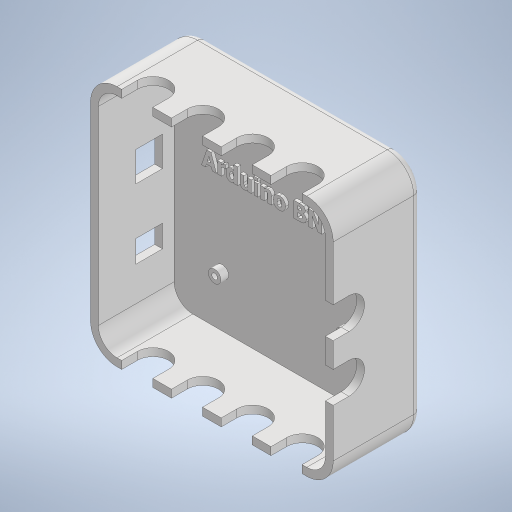
# Autodesk Inventor part: arduino_bnc_case_bottom
Saved by Autodesk Inventor 2024 (Build 280153000, 153)
## iProperties
Created: 2023-07-25
Part Number: arduino_bnc_case_bottom
Material: Generic
Document SubType Name: Modeling
Designer: maimon
Density: 1 g/cm^3
Appearance: Default
Author: maimon
Autodesk Inventor part; units mm, degrees
ref_plane "YZ Plane" through (0, 0, 0) normal (1, 0, 0) x (0, 1, 0)
ref_plane "XZ Plane" through (0, 0, 0) normal (0, 1, 0) x (-1, 0, 0)
ref_plane "XY Plane" through (0, 0, 0) normal (0, 0, 1) x (1, 0, 0)
sketch "Sketch1" plane through (0, 0, 0) normal (0, 0, 1) x (1, 0, 0)
  line L0 (-38.735, -46.355) -> (38.735, -46.355)
  line L1 (46.355, -38.735) -> (46.355, 38.735)
  line L2 (38.735, 46.355) -> (-38.735, 46.355)
  line L3 (-46.355, 38.735) -> (-46.355, -38.735)
  line L4 (-46.355, -46.355) -> (46.355, 46.355) construction
  line L5 (46.355, -46.355) -> (-46.355, 46.355) construction
  arc A0 (-38.735, 46.355) -> (-46.355, 38.735) centre (-38.735, 38.735) ccw
  arc A1 (-46.355, -38.735) -> (-38.735, -46.355) centre (-38.735, -38.735) ccw
  arc A2 (38.735, -46.355) -> (46.355, -38.735) centre (38.735, -38.735) ccw
  arc A3 (46.355, 38.735) -> (38.735, 46.355) centre (38.735, 38.735) ccw
  line L6 (38.735, -49.53) -> (-38.735, -49.53)
  arc A4 (-49.53, -38.735) -> (-38.735, -49.53) centre (-38.735, -38.735) ccw
  line L7 (-49.53, -38.735) -> (-49.53, 38.735)
  arc A5 (-38.735, 49.53) -> (-49.53, 38.735) centre (-38.735, 38.735) ccw
  line L8 (-38.735, 49.53) -> (38.735, 49.53)
  arc A6 (49.53, 38.735) -> (38.735, 49.53) centre (38.735, 38.735) ccw
  line L9 (49.53, 38.735) -> (49.53, -38.735)
  arc A7 (38.735, -49.53) -> (49.53, -38.735) centre (38.735, -38.735) ccw
  point P0 (0, 0)
  dimension "d0" = 92.71
  dimension "d1" = 92.71
  dimension "d3" = 7.62
  dimension "thick" = 3.175
  constraints: 20 end point, 16 point on circle, 8 centre point, 8 point on line, 8 tangent, 4 parallel, 3 equal radius, 2 midpoint, 2 perpendicular, 1 horizontal, 7 other
  measures "d0" distance of L5.end L4.end
  measures "d1" distance of L4.end L5.start
  measures "d3" radius of A0
  measures "thick" distance between parallel lines of L0 L6
extrude "Extrusion1" add sketch "Sketch1" along normal blind 30.95
sketch "Sketch2" plane through (0, 0, 0) normal (0, 0, -1) x (-1, 0, 0)
  line L0 (-38.735, 49.53) -> (38.735, 49.53) projected
  arc A0 (-38.735, 49.53) -> (-49.53, 38.735) centre (-38.735, 38.735) ccw projected
  line L1 (-49.53, -38.735) -> (-49.53, 38.735) projected
  arc A1 (-49.53, -38.735) -> (-38.735, -49.53) centre (-38.735, -38.735) ccw projected
  line L2 (38.735, -49.53) -> (-38.735, -49.53) projected
  arc A2 (38.735, -49.53) -> (49.53, -38.735) centre (38.735, -38.735) ccw projected
  line L3 (49.53, 38.735) -> (49.53, -38.735) projected
  arc A3 (49.53, 38.735) -> (38.735, 49.53) centre (38.735, 38.735) ccw projected
  arc A4 (38.735, -46.355) -> (46.355, -38.735) centre (38.735, -38.735) ccw projected
  line L4 (-38.735, -46.355) -> (38.735, -46.355) projected
  arc A5 (-46.355, -38.735) -> (-38.735, -46.355) centre (-38.735, -38.735) ccw projected
  line L5 (-46.355, 38.735) -> (-46.355, -38.735) projected
  arc A6 (-38.735, 46.355) -> (-46.355, 38.735) centre (-38.735, 38.735) ccw projected
  line L6 (38.735, 46.355) -> (-38.735, 46.355) projected
  arc A7 (46.355, 38.735) -> (38.735, 46.355) centre (38.735, 38.735) ccw projected
  line L7 (46.355, -38.735) -> (46.355, 38.735) projected
  point P0 (0, 0)
extrude "Extrusion2" add sketch "Sketch2" along normal blind 5.08 contours L0 A3 L3 A2 L2 A1 L1 A0 | L4 A5 L5 A6 L6 A7 L7 A4
sketch "Sketch3" plane through (0, 0, 0) normal (0, 0, 1) x (1, 0, 0)
  circle A0 centre (-26.67, -25.4) radius 2.54
  circle A1 centre (25.4, -20.28) radius 2.54
  circle A2 centre (25.4, 7.62) radius 2.54
  circle A3 centre (-25.4, 22.86) radius 2.54
  line L0 (38.735, -46.355) -> (-38.735, -46.355) projected
  line L1 (-46.355, -38.735) -> (-46.355, 38.735) projected
  line L2 (-38.735, 46.355) -> (38.735, 46.355) projected
  line L3 (46.355, 38.735) -> (46.355, -38.735) projected
  point P0 (0, 0)
  dimension "post_d" = 5.08
  dimension "d10" = 5.08
  dimension "d11" = 5.08
  dimension "d12" = 5.08
  dimension "d13" = 20.955
  dimension "d14" = 19.685
  dimension "d15" = 23.495
  dimension "d16" = 20.955
  dimension "d17" = 20.955
  dimension "d18" = 38.735
  dimension "d19" = 27.9
  constraints: 4 centre point, 1 vertical alignment
  measures "post_d" diameter of A0
  measures "d10" diameter of A3
  measures "d11" diameter of A2
  measures "d12" diameter of A1
  measures "d13" distance from line of L0 A0.centre
  measures "d14" distance from line of L1 A0.centre
  measures "d15" distance from line of L2 A3.centre
  measures "d16" distance from line of L1 A3.centre
  measures "d17" distance from line of A2.centre L3
  measures "d18" distance from line of L2 A2.centre
  measures "d19" distance of A1.centre A2.centre
extrude "Extrusion3" add sketch "Sketch3" along normal blind 3.175
sketch "Sketch4" plane through (25.4, -20.28, 3.175) normal (0, 0, 1) x (1, 0, 0)
  circle A0 centre (0, 0) radius 2.54 projected
  circle A1 centre (0, 0) radius 1.4224
  point P0 (-25.4, 20.28)
  dimension "d22" = 2.8448
  constraints: 1 centre point, 1 coincident
  measures "d22" diameter of A1
extrude "Extrusion4" add sketch "Sketch4" along normal blind 3.175 contours A1
sketch "Sketch5" plane through (-25.4, 22.86, 3.175) normal (0, 0, 1) x (1, 0, 0)
  circle A0 centre (0, 0) radius 2.54 projected
  circle A1 centre (-1.27, -48.26) radius 2.54 projected
  circle A2 centre (50.8, -15.24) radius 2.54 projected
  point P0 (25.4, -22.86)
  constraints: 3 coincident
hole "Hole1" at (-25.4, 22.86, 3.175) at (25.4, 7.62, 3.175) at (-26.67, -25.4, 3.175) direction (0, 0, -1) diameter 2.2606 end through all
sketch "Sketch6" plane through (-38.735, -49.53, 30.95) normal (0, -1, 0) x (1, 0, 0)
  line L0 (-7.62, -30.95) -> (-7.62, 0) projected
  line L1 (-7.62, -30.95) -> (-7.62, 0) projected
  line L2 (77.47, 0) -> (0, 0) projected
  line L3 (1.905, -6.439) -> (14.605, -6.439)
  line L4 (14.605, -6.439) -> (14.605, 0)
  line L5 (14.605, 0) -> (1.905, 0)
  line L6 (1.905, 0) -> (1.905, -6.439)
  line L7 (1.905, -6.439) -> (14.605, 0) construction
  line L8 (14.605, -6.439) -> (1.905, 0) construction
  arc A0 (1.905, -6.439) -> (14.605, -6.439) centre (8.255, -6.439) ccw
  line L9 (61.595, -30.95) -> (66.675, -30.95) projected
  line L10 (10.795, -30.95) -> (15.875, -30.95) projected
  line L11 (61.595, -30.95) -> (66.675, -30.95) projected
  line L12 (9.525, -30.95) -> (14.605, -30.95) projected
  line L13 (77.47, -30.95) -> (0, -30.95) projected
  line L14 (85.09, -30.95) -> (77.47, -30.95) projected
  line L15 (77.47, -30.95) -> (85.09, -30.95) projected
  line L16 (0, -30.95) -> (77.47, -30.95) projected
  line L17 (-7.62, -30.95) -> (0, -30.95) projected
  line L18 (0, -30.95) -> (-7.62, -30.95) projected
  point P0 (38.735, -30.95)
  point P1 (8.255, -3.2195)
  point P2 (8.255, -12.789)
  point P3 (1.905, 0)
  dimension "d32" = 15.875
  dimension "bnc_d" = 12.7
  dimension "bnc_h" = 18.161
  dimension "d36" = 12.789
  constraints: 12 end point, 3 point on circle, 2 midpoint, 2 parallel, 2 tangent, 1 centre point, 1 horizontal, 1 perpendicular, 1 point on line
  measures "d32" distance from line of L0 point (8.255, -3.219)
  measures "bnc_d" distance between parallel lines of L4 L6
  measures "bnc_h" distance from line of L13 point (8.255, -12.789)
  measures "d36" distance from line of L2 point (8.255, -12.789)
extrude "Extrusion5" cut sketch "Sketch6" against normal up to surface (99.06 mm away)
pattern_linear "Rectangular Pattern1" count 4 spacing 20.32 along (1, 0, 0) of "Extrusion5"
sketch "Sketch7" plane through (49.53, -38.735, 30.95) normal (1, 0, 0) x (0, 0, -1)
  line L0 (0, -7.62) -> (6.439, -7.62) projected
  line L1 (6.439, -7.62) -> (6.439, -7.62) projected
  line L2 (6.439, -7.62) -> (0, -7.62) projected
  line L3 (30.95, -7.62) -> (0, -7.62) projected
  line L4 (30.95, -7.62) -> (0, -7.62) projected
  line L5 (0, -7.62) -> (6.439, -7.62) projected
  line L6 (6.439, -7.62) -> (6.439, -7.62) projected
  line L7 (6.439, -7.62) -> (0, -7.62) projected
  line L8 (0, -7.62) -> (6.439, -7.62) projected
  line L9 (6.439, -7.62) -> (6.439, -7.62) projected
  line L10 (6.439, -7.62) -> (0, -7.62) projected
  line L11 (0, -7.62) -> (6.439, -7.62) projected
  line L12 (6.439, -7.62) -> (6.439, -7.62) projected
  line L13 (6.439, -7.62) -> (0, -7.62) projected
  line L14 (30.95, 43.815) -> (30.95, 48.895) projected
  line L15 (30.95, 59.055) -> (30.95, 64.135) projected
  line L16 (30.95, 15.915) -> (30.95, 20.995) projected
  line L17 (30.95, 10.795) -> (30.95, 15.875) projected
  line L18 (30.95, 0) -> (30.95, -7.62) projected
  line L19 (30.95, 77.47) -> (30.95, 0) projected
  line L20 (30.95, 85.09) -> (30.95, 77.47) projected
  line L21 (30.95, 77.47) -> (30.95, 85.09) projected
  line L22 (30.95, 0) -> (30.95, 77.47) projected
  line L23 (30.95, -7.62) -> (30.95, 0) projected
  line L24 (0, 77.47) -> (0, 0) projected
  line L25 (6.439, 19.685) -> (0, 19.685)
  line L26 (0, 19.685) -> (0, 32.385)
  line L27 (0, 32.385) -> (6.439, 32.385)
  line L28 (6.439, 32.385) -> (6.439, 19.685)
  line L29 (6.439, 19.685) -> (0, 32.385) construction
  line L30 (0, 19.685) -> (6.439, 32.385) construction
  arc A0 (6.439, 19.685) -> (6.439, 32.385) centre (6.439, 26.035) ccw
  point P0 (30.95, 38.735)
  point P1 (3.2195, 26.035)
  point P2 (12.789, 26.035)
  point P3 (0, 19.685)
  dimension "d42" = 12.7
  dimension "d43" = 18.161
  dimension "d44" = 33.655
  constraints: 12 end point, 3 point on circle, 2 midpoint, 2 parallel, 2 tangent, 1 centre point, 1 horizontal, 1 perpendicular, 1 point on line
  measures "d42" distance between parallel lines of L27 L25
  measures "d43" distance from line of point (12.789, 26.035) L19
  measures "d44" distance from line of L3 point (3.219, 26.035)
extrude "Extrusion6" cut sketch "Sketch7" against normal up to next
pattern_linear "Rectangular Pattern2" count 2 spacing 22.86 along (0, 1, 0) of "Extrusion6"
sketch "Sketch8" plane through (-49.53, -38.735, 30.95) normal (-1, 0, 0) x (0, 0, 1)
  line L0 (-27.775, 62.7253) -> (-27.775, 60.4647) projected
  line L1 (-36.03, 60.4647) -> (-36.03, 62.7253) projected
  line L2 (-27.775, 62.7253) -> (-27.775, 60.4647) projected
  line L3 (-36.03, 12.2047) -> (-36.03, 14.4653) projected
  line L4 (-27.775, 14.4653) -> (-27.775, 12.2047) projected
  line L5 (0, -7.62) -> (-6.439, -7.62) projected
  line L6 (-6.439, -7.62) -> (-6.439, -7.62) projected
  line L7 (-6.439, -7.62) -> (0, -7.62) projected
  line L8 (-30.95, -7.62) -> (0, -7.62) projected
  line L9 (-30.95, -7.62) -> (0, -7.62) projected
  line L10 (0, -7.62) -> (-6.439, -7.62) projected
  line L11 (-6.439, -7.62) -> (-6.439, -7.62) projected
  line L12 (-6.439, -7.62) -> (0, -7.62) projected
  line L13 (0, -7.62) -> (-6.439, -7.62) projected
  line L14 (-6.439, -7.62) -> (-6.439, -7.62) projected
  line L15 (-6.439, -7.62) -> (0, -7.62) projected
  line L16 (0, -7.62) -> (-6.439, -7.62) projected
  line L17 (-6.439, -7.62) -> (-6.439, -7.62) projected
  line L18 (-6.439, -7.62) -> (0, -7.62) projected
  line L19 (-6.439, 85.09) -> (0, 85.09) projected
  line L20 (0, 85.09) -> (-6.439, 85.09) projected
  line L21 (-6.439, 85.09) -> (-6.439, 85.09) projected
  line L22 (-6.439, 85.09) -> (0, 85.09) projected
  line L23 (0, 85.09) -> (-6.439, 85.09) projected
  line L24 (-6.439, 85.09) -> (-6.439, 85.09) projected
  line L25 (-6.439, 85.09) -> (0, 85.09) projected
  line L26 (0, 85.09) -> (-6.439, 85.09) projected
  line L27 (-6.439, 85.09) -> (-6.439, 85.09) projected
  line L28 (-6.439, 85.09) -> (0, 85.09) projected
  line L29 (-30.95, 85.09) -> (0, 85.09) projected
  line L30 (-30.95, 85.09) -> (0, 85.09) projected
  line L31 (0, 85.09) -> (-6.439, 85.09) projected
  line L32 (-6.439, 85.09) -> (-6.439, 85.09) projected
  line L33 (-27.775, 10.795) -> (-26.175, 10.795) construction
  line L34 (-26.175, 10.795) -> (-26.175, 64.095) construction
  line L35 (-26.175, 64.095) -> (-27.775, 64.095) construction
  line L36 (-27.775, 64.095) -> (-27.775, 10.795) construction
  line L37 (-26.175, 13.995) -> (-15.275, 13.995)
  line L38 (-15.275, 13.995) -> (-15.275, 23.095)
  line L39 (-15.275, 23.095) -> (-26.175, 23.095)
  line L40 (-26.175, 23.095) -> (-26.175, 13.995)
  line L41 (-26.175, 42.395) -> (-15.275, 42.395)
  line L42 (-15.275, 42.395) -> (-15.275, 54.595)
  line L43 (-15.275, 54.595) -> (-26.175, 54.595)
  line L44 (-26.175, 54.595) -> (-26.175, 42.395)
  point P0 (-30.95, 38.735)
  point P1 (-27.775, 13.335)
  point P2 (-27.775, 61.595)
  point P3 (-26.975, 10.795)
  point P4 (-26.975, 64.095)
  dimension "d50" = 53.3
  dimension "d51" = 1.6
  dimension "d53" = 2.5
  dimension "d54" = 18.415
  dimension "d55" = 2.54
  dimension "d56" = 10.9
  dimension "d57" = 9.1
  dimension "d58" = 12.2
  dimension "d59" = 9.5
  dimension "d60" = 3.2
  constraints: 24 end point, 6 parallel, 4 midpoint, 3 horizontal, 3 perpendicular, 3 point on line, 1 vertical alignment
  measures "d50" distance of L33.end L34.end
  measures "d51" distance between parallel lines of L34 L36
  measures "d53" distance from line of L35 point (-27.775, 61.595)
  measures "d54" distance between parallel lines of L8 L33
  measures "d55" vertical distance of point (-26.975, 10.795) point (-27.775, 13.335)
  measures "d56" distance of L39.end L38.end
  measures "d57" distance of L38.end L37.end
  measures "d58" distance of L41.end L42.end
  measures "d59" distance from line of point (-26.975, 64.095) L43
  measures "d60" distance between parallel lines of L33 L37
extrude "Extrusion7" cut sketch "Sketch8" against normal up to next
fillet "Fillet1" radius 3.175 8 edges at (-46.3682, -46.3682, -5.08) (-49.53, 0, -5.08) (-46.3682, 46.3682, -5.08) (0, 49.53, -5.08) (46.3682, 46.3682, -5.08) (49.53, 0, -5.08) (46.3682, -46.3682, -5.08) (0, -49.53, -5.08)
sketch "Sketch9" plane through (0, 0, 0) normal (0, 0, 1) x (1, 0, 0)
  line L0 (-33.8863, 16.1091) -> (28.0046, 16.1091) construction
  line L1 (28.0046, 16.1091) -> (28.0046, -6.8386) construction
  line L2 (28.0046, -6.8386) -> (-33.8863, -6.8386) construction
  line L3 (-33.8863, -6.8386) -> (-33.8863, 16.1091) construction
  line L4 (-33.912, 9.471) -> (-31.7662, 15.821)
  line L5 (-31.7662, 15.821) -> (-30.0269, 15.821)
  line L6 (-30.0269, 15.821) -> (-27.8811, 9.471)
  line L7 (-27.8811, 9.471) -> (-29.5226, 9.471)
  line L8 (-29.5226, 9.471) -> (-29.9188, 10.7677)
  line L9 (-29.9188, 10.7677) -> (-31.9154, 10.7677)
  line L10 (-31.9154, 10.7677) -> (-32.3168, 9.471)
  line L11 (-32.3168, 9.471) -> (-33.912, 9.471)
  line L12 (-30.2688, 11.9204) -> (-30.9171, 14.0199)
  line L13 (-30.9171, 14.0199) -> (-31.5707, 11.9204)
  line L14 (-31.5707, 11.9204) -> (-30.2688, 11.9204)
  line L15 (-24.1194, 12.8467) -> (-24.2429, 12.8467)
  spline S0 degree 2 poles (-24.2429, 12.8467) (-24.3304, 12.8775) (-24.6546, 12.9084) (-24.8502, 12.9084) knots 0 0 0 1 2 2 2
  spline S1 degree 2 poles (-24.8502, 12.9084) (-25.0817, 12.9084) (-25.6015, 12.7695) (-25.8433, 12.6768) knots 0 0 0 1 2 2 2
  line L16 (-25.8433, 12.6768) -> (-25.8433, 9.471)
  line L17 (-25.8433, 9.471) -> (-27.3356, 9.471)
  line L18 (-27.3356, 9.471) -> (-27.3356, 14.2618)
  line L19 (-27.3356, 14.2618) -> (-25.8433, 14.2618)
  line L20 (-25.8433, 14.2618) -> (-25.8433, 13.5722)
  spline S2 degree 2 poles (-25.8433, 13.5722) (-25.7404, 13.6649) (-25.3802, 13.953) (-25.231, 14.0405) knots 0 0 0 1 2 2 2
  spline S3 degree 2 poles (-25.231, 14.0405) (-25.0663, 14.1383) (-24.634, 14.2772) (-24.4436, 14.2772) knots 0 0 0 1 2 2 2
  spline S4 degree 2 poles (-24.4436, 14.2772) (-24.3716, 14.2772) (-24.1915, 14.2669) (-24.1194, 14.2618) knots 0 0 0 1 2 2 2
  line L21 (-24.1194, 14.2618) -> (-24.1194, 12.8467)
  line L22 (-19.1949, 9.471) -> (-20.6872, 9.471)
  line L23 (-20.6872, 9.471) -> (-20.6872, 9.9701)
  spline S5 degree 2 poles (-20.6872, 9.9701) (-20.8312, 9.8518) (-21.2017, 9.579) (-21.3458, 9.507) knots 0 0 0 1 2 2 2
  spline S6 degree 2 poles (-21.3458, 9.507) (-21.5208, 9.4247) (-21.8707, 9.3372) (-22.1126, 9.3372) knots 0 0 0 1 2 2 2
  spline S7 degree 2 poles (-22.1126, 9.3372) (-22.9308, 9.3372) (-23.8879, 10.6957) (-23.8879, 11.8278) knots 0 0 0 1 2 2 2
  spline S8 degree 2 poles (-23.8879, 11.8278) (-23.8879, 12.4556) (-23.5637, 13.3767) (-23.2807, 13.7163) knots 0 0 0 1 2 2 2
  spline S9 degree 2 poles (-23.2807, 13.7163) (-23.0182, 14.0302) (-22.2772, 14.3904) (-21.8656, 14.3904) knots 0 0 0 1 2 2 2
  spline S10 degree 2 poles (-21.8656, 14.3904) (-21.4899, 14.3904) (-21.0062, 14.2309) (-20.6872, 14.0662) knots 0 0 0 1 2 2 2
  line L24 (-20.6872, 14.0662) -> (-20.6872, 16.104)
  line L25 (-20.6872, 16.104) -> (-19.1949, 16.104)
  line L26 (-19.1949, 16.104) -> (-19.1949, 9.471)
  line L27 (-20.6872, 10.7883) -> (-20.6872, 13.14)
  spline S11 degree 2 poles (-20.6872, 13.14) (-20.7952, 13.1966) (-21.1554, 13.2686) (-21.2841, 13.2686) knots 0 0 0 1 2 2 2
  spline S12 degree 2 poles (-21.2841, 13.2686) (-21.8192, 13.2686) (-22.3596, 12.5173) (-22.3596, 11.8432) knots 0 0 0 1 2 2 2
  spline S13 degree 2 poles (-22.3596, 11.8432) (-22.3596, 11.1331) (-21.9273, 10.5001) (-21.4487, 10.5001) knots 0 0 0 1 2 2 2
  spline S14 degree 2 poles (-21.4487, 10.5001) (-21.2532, 10.5001) (-20.8518, 10.6545) (-20.6872, 10.7883) knots 0 0 0 1 2 2 2
  line L28 (-13.6064, 9.471) -> (-15.0987, 9.471)
  line L29 (-15.0987, 9.471) -> (-15.0987, 10.001)
  spline S15 degree 2 poles (-15.0987, 10.001) (-15.4847, 9.6768) (-16.1331, 9.3372) (-16.5808, 9.3372) knots 0 0 0 1 2 2 2
  spline S16 degree 2 poles (-16.5808, 9.3372) (-17.2909, 9.3372) (-18.0885, 10.2377) (-18.0885, 11.1434) knots 0 0 0 1 2 2 2
  line L30 (-18.0885, 11.1434) -> (-18.0885, 14.2618)
  line L31 (-18.0885, 14.2618) -> (-16.5859, 14.2618)
  line L32 (-16.5859, 14.2618) -> (-16.5859, 11.8844)
  spline S17 degree 2 poles (-16.5859, 11.8844) (-16.5859, 11.5139) (-16.5499, 11.0405) (-16.4778, 10.8809) knots 0 0 0 1 2 2 2
  spline S18 degree 2 poles (-16.4778, 10.8809) (-16.4058, 10.7317) (-16.1228, 10.5773) (-15.8655, 10.5773) knots 0 0 0 1 2 2 2
  spline S19 degree 2 poles (-15.8655, 10.5773) (-15.7111, 10.5773) (-15.2788, 10.7317) (-15.0987, 10.8655) knots 0 0 0 1 2 2 2
  line L33 (-15.0987, 10.8655) -> (-15.0987, 14.2618)
  line L34 (-15.0987, 14.2618) -> (-13.6064, 14.2618)
  line L35 (-13.6064, 14.2618) -> (-13.6064, 9.471)
  line L36 (-10.9718, 9.471) -> (-12.4641, 9.471)
  line L37 (-12.4641, 9.471) -> (-12.4641, 14.2618)
  line L38 (-12.4641, 14.2618) -> (-10.9718, 14.2618)
  line L39 (-10.9718, 14.2618) -> (-10.9718, 9.471)
  line L40 (-10.9254, 14.9462) -> (-12.5052, 14.9462)
  line L41 (-12.5052, 14.9462) -> (-12.5052, 16.1091)
  line L42 (-12.5052, 16.1091) -> (-10.9254, 16.1091)
  line L43 (-10.9254, 16.1091) -> (-10.9254, 14.9462)
  line L44 (-5.3473, 9.471) -> (-6.8499, 9.471)
  line L45 (-6.8499, 9.471) -> (-6.8499, 11.8432)
  spline S20 degree 2 poles (-6.8499, 11.8432) (-6.8499, 12.1365) (-6.8962, 12.7129) (-6.958, 12.8467) knots 0 0 0 1 2 2 2
  spline S21 degree 2 poles (-6.958, 12.8467) (-7.0352, 13.0113) (-7.3233, 13.1503) (-7.5703, 13.1503) knots 0 0 0 1 2 2 2
  spline S22 degree 2 poles (-7.5703, 13.1503) (-7.7504, 13.1503) (-8.1261, 13.0113) (-8.3371, 12.8621) knots 0 0 0 1 2 2 2
  line L46 (-8.3371, 12.8621) -> (-8.3371, 9.471)
  line L47 (-8.3371, 9.471) -> (-9.8294, 9.471)
  line L48 (-9.8294, 9.471) -> (-9.8294, 14.2618)
  line L49 (-9.8294, 14.2618) -> (-8.3371, 14.2618)
  line L50 (-8.3371, 14.2618) -> (-8.3371, 13.7318)
  spline S23 degree 2 poles (-8.3371, 13.7318) (-7.9717, 14.0405) (-7.277, 14.3904) (-6.8551, 14.3904) knots 0 0 0 1 2 2 2
  spline S24 degree 2 poles (-6.8551, 14.3904) (-6.1243, 14.3904) (-5.3473, 13.4642) (-5.3473, 12.5894) knots 0 0 0 1 2 2 2
  line L51 (-5.3473, 12.5894) -> (-5.3473, 9.471)
  spline S25 degree 2 poles (0.3543, 11.8638) (0.3543, 10.6803) (-0.9373, 9.3217) (-2.1157, 9.3217) knots 0 0 0 1 2 2 2
  spline S26 degree 2 poles (-2.1157, 9.3217) (-3.289, 9.3217) (-4.5909, 10.6803) (-4.5909, 11.8638) knots 0 0 0 1 2 2 2
  spline S27 degree 2 poles (-4.5909, 11.8638) (-4.5909, 13.0576) (-3.289, 14.411) (-2.1157, 14.411) knots 0 0 0 1 2 2 2
  spline S28 degree 2 poles (-2.1157, 14.411) (-0.9425, 14.411) (0.3543, 13.0525) (0.3543, 11.8638) knots 0 0 0 1 2 2 2
  spline S29 degree 2 poles (-1.174, 11.8535) (-1.174, 12.2806) (-1.313, 12.8518) (-1.4365, 13.0216) knots 0 0 0 1 2 2 2
  spline S30 degree 2 poles (-1.4365, 13.0216) (-1.5703, 13.2017) (-1.9047, 13.3407) (-2.1157, 13.3407) knots 0 0 0 1 2 2 2
  spline S31 degree 2 poles (-2.1157, 13.3407) (-2.3216, 13.3407) (-2.6457, 13.2172) (-2.7795, 13.0422) knots 0 0 0 1 2 2 2
  spline S32 degree 2 poles (-2.7795, 13.0422) (-2.9082, 12.8775) (-3.0626, 12.2961) (-3.0626, 11.8535) knots 0 0 0 1 2 2 2
  spline S33 degree 2 poles (-3.0626, 11.8535) (-3.0626, 11.4161) (-2.9185, 10.8758) (-2.8001, 10.7111) knots 0 0 0 1 2 2 2
  spline S34 degree 2 poles (-2.8001, 10.7111) (-2.6818, 10.5465) (-2.3216, 10.3921) (-2.1054, 10.3921) knots 0 0 0 1 2 2 2
  spline S35 degree 2 poles (-2.1054, 10.3921) (-1.9253, 10.3921) (-1.5548, 10.5465) (-1.4416, 10.7008) knots 0 0 0 1 2 2 2
  spline S36 degree 2 poles (-1.4416, 10.7008) (-1.313, 10.8809) (-1.174, 11.4007) (-1.174, 11.8535) knots 0 0 0 1 2 2 2
  spline S37 degree 2 poles (8.8656, 11.4161) (8.8656, 10.9427) (8.5054, 10.2274) (8.2069, 9.9907) knots 0 0 0 1 2 2 2
  spline S38 degree 2 poles (8.2069, 9.9907) (7.8467, 9.7077) (6.9925, 9.471) (6.3286, 9.471) knots 0 0 0 1 2 2 2
  line L52 (6.3286, 9.471) -> (3.7917, 9.471)
  line L53 (3.7917, 9.471) -> (3.7917, 15.821)
  line L54 (3.7917, 15.821) -> (6.0302, 15.821)
  spline S39 degree 2 poles (6.0302, 15.821) (6.73, 15.821) (7.4504, 15.7129) (7.7643, 15.5431) knots 0 0 0 1 2 2 2
  spline S40 degree 2 poles (7.7643, 15.5431) (8.1091, 15.363) (8.4436, 14.7455) (8.4436, 14.3441) knots 0 0 0 1 2 2 2
  spline S41 degree 2 poles (8.4436, 14.3441) (8.4436, 13.881) (7.9805, 13.1554) (7.5688, 12.9856) knots 0 0 0 1 2 2 2
  line L55 (7.5688, 12.9856) -> (7.5688, 12.9547)
  spline S42 degree 2 poles (7.5688, 12.9547) (8.1606, 12.8312) (8.8656, 12.0645) (8.8656, 11.4161) knots 0 0 0 1 2 2 2
  spline S43 degree 2 poles (7.2189, 11.4418) (7.2189, 11.7403) (6.9822, 12.0748) (6.7455, 12.1623) knots 0 0 0 1 2 2 2
  spline S44 degree 2 poles (6.7455, 12.1623) (6.6014, 12.2189) (6.0919, 12.2292) (5.67, 12.2292) knots 0 0 0 1 2 2 2
  line L56 (5.67, 12.2292) -> (5.3767, 12.2292)
  line L57 (5.3767, 12.2292) -> (5.3767, 10.6288)
  line L58 (5.3767, 10.6288) -> (5.4641, 10.6288)
  spline S45 degree 2 poles (5.4641, 10.6288) (6.0816, 10.6288) (6.5551, 10.6442) (6.8021, 10.7523) knots 0 0 0 1 2 2 2
  spline S46 degree 2 poles (6.8021, 10.7523) (7.0182, 10.8501) (7.2189, 11.2103) (7.2189, 11.4418) knots 0 0 0 1 2 2 2
  spline S47 degree 2 poles (6.8227, 14.0302) (6.8227, 14.1846) (6.6631, 14.5088) (6.4985, 14.5808) knots 0 0 0 1 2 2 2
  spline S48 degree 2 poles (6.4985, 14.5808) (6.3441, 14.6529) (5.9118, 14.6632) (5.4847, 14.6632) knots 0 0 0 1 2 2 2
  line L59 (5.4847, 14.6632) -> (5.3767, 14.6632)
  line L60 (5.3767, 14.6632) -> (5.3767, 13.3149)
  line L61 (5.3767, 13.3149) -> (5.5774, 13.3149)
  spline S49 degree 2 poles (5.5774, 13.3149) (5.9839, 13.3149) (6.3132, 13.3304) (6.4882, 13.4127) knots 0 0 0 1 2 2 2
  spline S50 degree 2 poles (6.4882, 13.4127) (6.6786, 13.5053) (6.8227, 13.8192) (6.8227, 14.0302) knots 0 0 0 1 2 2 2
  line L62 (15.2207, 9.471) -> (13.6872, 9.471)
  line L63 (13.6872, 9.471) -> (11.2378, 13.8964)
  line L64 (11.2378, 13.8964) -> (11.2378, 9.471)
  line L65 (11.2378, 9.471) -> (9.7815, 9.471)
  line L66 (9.7815, 9.471) -> (9.7815, 15.821)
  line L67 (9.7815, 15.821) -> (11.737, 15.821)
  line L68 (11.737, 15.821) -> (13.7644, 12.1828)
  line L69 (13.7644, 12.1828) -> (13.7644, 15.821)
  line L70 (13.7644, 15.821) -> (15.2207, 15.821)
  line L71 (15.2207, 15.821) -> (15.2207, 9.471)
  spline S51 degree 2 poles (19.2499, 9.3475) (17.8194, 9.3475) (16.1418, 11.0765) (16.1418, 12.6408) knots 0 0 0 1 2 2 2
  spline S52 degree 2 poles (16.1418, 12.6408) (16.1418, 14.1486) (17.8245, 15.9445) (19.2551, 15.9445) knots 0 0 0 1 2 2 2
  spline S53 degree 2 poles (19.2551, 15.9445) (19.6307, 15.9445) (20.2379, 15.857) (20.5158, 15.785) knots 0 0 0 1 2 2 2
  spline S54 degree 2 poles (20.5158, 15.785) (20.7319, 15.7181) (21.2414, 15.4968) (21.4009, 15.4144) knots 0 0 0 1 2 2 2
  line L72 (21.4009, 15.4144) -> (21.4009, 13.9016)
  line L73 (21.4009, 13.9016) -> (21.2414, 13.9016)
  spline S55 degree 2 poles (21.2414, 13.9016) (21.123, 14.0045) (20.7731, 14.2927) (20.5518, 14.4264) knots 0 0 0 1 2 2 2
  spline S56 degree 2 poles (20.5518, 14.4264) (20.3306, 14.5654) (19.8005, 14.7558) (19.5072, 14.7558) knots 0 0 0 1 2 2 2
  spline S57 degree 2 poles (19.5072, 14.7558) (19.1624, 14.7558) (18.5912, 14.5397) (18.3288, 14.2669) knots 0 0 0 1 2 2 2
  spline S58 degree 2 poles (18.3288, 14.2669) (18.0921, 14.0251) (17.7885, 13.1966) (17.7885, 12.6357) knots 0 0 0 1 2 2 2
  spline S59 degree 2 poles (17.7885, 12.6357) (17.7885, 12.0439) (18.1024, 11.236) (18.3597, 10.989) knots 0 0 0 1 2 2 2
  spline S60 degree 2 poles (18.3597, 10.989) (18.6067, 10.7471) (19.2139, 10.5362) (19.5175, 10.5362) knots 0 0 0 1 2 2 2
  spline S61 degree 2 poles (19.5175, 10.5362) (19.8314, 10.5362) (20.4026, 10.7471) (20.5981, 10.8758) knots 0 0 0 1 2 2 2
  spline S62 degree 2 poles (20.5981, 10.8758) (20.8143, 11.0044) (21.1385, 11.2772) (21.2568, 11.3852) knots 0 0 0 1 2 2 2
  line L74 (21.2568, 11.3852) -> (21.4009, 11.3852)
  line L75 (21.4009, 11.3852) -> (21.4009, 9.8929)
  spline S63 degree 2 poles (21.4009, 9.8929) (21.2259, 9.8106) (20.768, 9.6048) (20.5209, 9.5327) knots 0 0 0 1 2 2 2
  spline S64 degree 2 poles (20.5209, 9.5327) (20.2225, 9.4401) (19.7028, 9.3475) (19.2499, 9.3475) knots 0 0 0 1 2 2 2
  point P0 (0, 0)
  constraints: 2 other
emboss "Emboss1" sketch "Sketch9" operation add depth 1.27 direction (0, 0, -1)
equation "\"d10\" = post_d"
equation "\"d11\" = post_d"
equation "\"d12\" = post_d"
equation "\"d42\" = bnc_d"
equation "\"d43\" = bnc_h"
equation "\"tol\" = 0.635"
body "Solid1"
